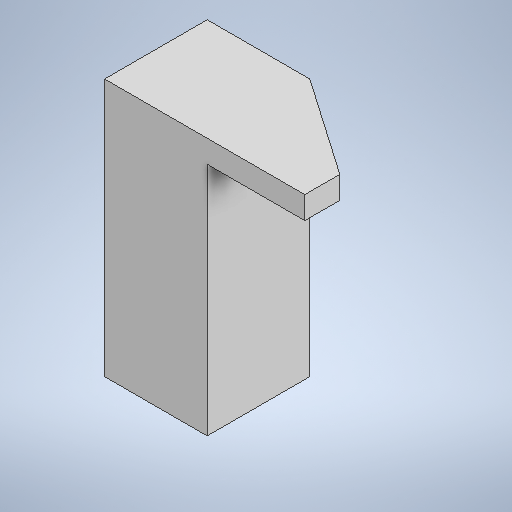
# Autodesk Inventor part: Pata2
Saved by Autodesk Inventor 2025 (Build 290162000, 162)
## iProperties
Created: 2026-09-16
Part Number: Pata2
Material: Genérico
Document SubType Name: Modeling
Designer: ASUS
Density: 1 g/cm^3
Appearance: Valor por defecto
Author: ASUS
Autodesk Inventor part; units mm, degrees
ref_plane "YZ Plane" through (0, 0, 0) normal (1, 0, 0) x (0, 1, 0)
ref_plane "XZ Plane" through (0, 0, 0) normal (0, 1, 0) x (-1, 0, 0)
ref_plane "XY Plane" through (0, 0, 0) normal (0, 0, 1) x (1, 0, 0)
sketch "Boceto1" plane through (0, 0, 0) normal (0, 1, 0) x (-1, 0, 0)
  line L0 (20.5, -20.5) -> (-20.5, -20.5)
  line L1 (-20.5, -20.5) -> (-20.5, 20.5)
  line L2 (-20.5, 20.5) -> (20.5, 20.5)
  line L3 (20.5, 20.5) -> (20.5, -20.5)
  point P0 (0, 0)
  point P1 (0, 20.5)
  point P2 (-20.5, 0)
  dimension "d0" = 41
  dimension "d1" = 41
  constraints: 8 end point, 2 midpoint, 2 parallel, 1 horizontal, 1 horizontal alignment, 1 perpendicular, 1 vertical alignment
  measures "d0" distance of L1.end L2.end
  measures "d1" distance of L0.end L1.end
extrude "Extrusión1" add sketch "Boceto1" along normal blind 94
sketch "Boceto2" plane through (0, 94, 0) normal (0, 1, 0) x (1, 0, 0)
  line L0 (-20.5, 20.5) -> (-20.5, -20.5) projected
  line L1 (-20.5, -20.5) -> (20.5, -20.5) projected
  line L2 (20.5, -20.5) -> (20.5, 20.5) projected
  line L3 (20.5, -20.5) -> (59.5, -20.5)
  line L4 (59.5, -20.5) -> (59.5, -6.5)
  line L5 (22.2539, -18.5) -> (57.5, -18.5)
  line L6 (57.5, -18.5) -> (22.5, -18.5)
  line L7 (22.5, -18.5) -> (22.5, -2.5)
  line L8 (57.5, -18.5) -> (57.5, -7.55)
  line L9 (22.5, -2.5) -> (50.21, -2.5)
  line L10 (22.5, -0.5) -> (47.32, -0.5)
  line L11 (22.5, -0.5) -> (22.5, 16.68)
  line L12 (22.5, 16.68) -> (47.32, -0.5)
  line L13 (50.21, -2.5) -> (57.5, -7.55)
  line L14 (20.5, 20.5) -> (-20.5, 20.5) projected
  line L15 (20.5, 20.5) -> (59.5, -6.5)
  point P0 (0, 0)
  dimension "d23" = 39
  dimension "d24" = 14
  dimension "d25" = 35
  dimension "d26" = 2
  dimension "d27" = 16
  dimension "d28" = 2
  dimension "d29" = 10.95
  dimension "d30" = 27.71
  dimension "d31" = 24.82
  dimension "d32" = 2
  dimension "d33" = 17.18
  constraints: 24 end point, 4 horizontal, 3 vertical, 1 perpendicular, 1 point on line
  measures "d23" distance of L1.end L3.end
  measures "d24" distance of L3.end L4.end
  measures "d25" distance of L5.end L6.end
  measures "d26" distance between parallel lines of L3 L5
  measures "d27" distance of L6.end L7.end
  measures "d28" distance between parallel lines of L2 L7
  measures "d29" distance of L5.end L8.end
  measures "d30" distance of L7.end L9.end
  measures "d31" distance of L10.start L10.end
  measures "d32" distance between parallel lines of L9 L10
  measures "d33" distance of L10.start L11.end
sketch "Boceto3" plane through (0, 94, 0) normal (0, 1, 0) x (1, 0, 0)
  point P0 (0, 0)
sketch "Boceto4" plane through (0, 94, 0) normal (0, 1, 0) x (1, 0, 0)
  point P0 (0, 0)
extrude "Extrusión2" add sketch "Boceto2" along normal blind 8 contours L15 L4 L3 L2
sketch "Boceto5" plane through (0, 94, 0) normal (0, 1, 0) x (1, 0, 0)
  line L0 (20.5, 20.5) -> (-20.5, 20.5) projected
  line L1 (-20.5, -20.5) -> (20.5, -20.5) projected
  line L2 (-20.5, 20.5) -> (20.5, 20.5)
  line L3 (20.5, 20.5) -> (20.5, -20.5)
  line L4 (20.5, -20.5) -> (-20.5, -20.5)
  line L5 (-20.5, -20.5) -> (-20.5, 20.5)
  point P0 (0, 0)
  constraints: 8 end point, 2 parallel, 1 horizontal, 1 perpendicular
extrude "Extrusión3" add sketch "Boceto5" along normal blind 8
sketch "Boceto7" plane through (0, 102, 0) normal (0, 1, 0) x (1, 0, 0)
  line L0 (20.5, 20.5) -> (-20.5, 20.5) projected
  line L1 (-20.5, 20.5) -> (20.5, 20.5)
  line L2 (59.5, -20.5) -> (59.5, -6.5) projected
  line L3 (20.5, 20.5) -> (59.5, -6.5)
  line L4 (59.5, -6.5) -> (59.5, -20.5)
  line L5 (59.5, -20.5) -> (-20.5, -20.5)
  line L6 (-20.5, -20.5) -> (-20.5, 20.5)
  point P0 (0, 0)
  constraints: 10 end point, 2 collinear, 2 perpendicular
extrude "Extrusión5" add sketch "Boceto7" along normal blind 1
